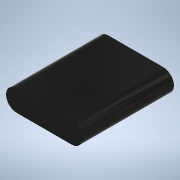
# Autodesk Inventor part: anker_battery_pack
Saved by Autodesk Inventor 2020.3 (Build 243373000, 373)
## iProperties
Created: 2020-07-01
Part Number: anker_battery_pack
Material: Generic
Document SubType Name: Modeling
Designer: Devin
Density: 1 g/cm^3
Appearance: Smooth - Black
Author: Devin
Autodesk Inventor part; units mm, degrees
ref_plane "YZ Plane" through (0, 0, 0) normal (1, 0, 0) x (0, 1, 0)
ref_plane "XZ Plane" through (0, 0, 0) normal (0, 1, 0) x (-1, 0, 0)
ref_plane "XY Plane" through (0, 0, 0) normal (0, 0, 1) x (1, 0, 0)
sketch "Sketch1" plane through (0, 0, 0) normal (0, 1, 0) x (-1, 0, 0)
  line L0 (0, 0) -> (0, -97.3)
  line L1 (0, -97.3) -> (-80.85, -97.3)
  line L2 (-80.85, -97.3) -> (-80.85, 0)
  line L3 (-80.85, 0) -> (0, 0)
  dimension "d0" = 97.3
  dimension "d1" = 80.85
  constraints: 8 end point, 2 parallel, 1 perpendicular, 1 vertical
  measures "d0" distance of L0.start L0.end
  measures "d1" distance of L0.end L1.end
extrude "Extrusion1" add sketch "Sketch1" along normal blind 22.5
fillet "Fillet2" radius 11.25 4 edges at (80.85, 22.5, -48.65) (0, 22.5, -48.65) (80.85, 0, -48.65) (0, 0, -48.65)
body "Solid1"
